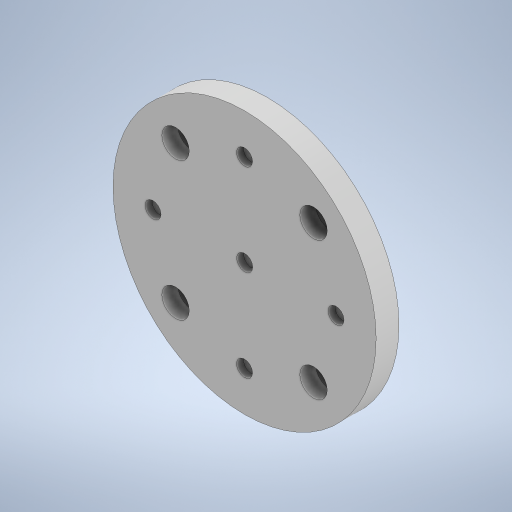
# Autodesk Inventor part: adaptor_spine_base
Saved by Autodesk Inventor 2024 (Build 280153000, 153)
## iProperties
Created: 2024-05-24
Part Number: adaptor_spine_base
Material: Generic
Document SubType Name: Modeling
Designer: maint
Density: 1 g/cm^3
Appearance: Default
Author: maint
Autodesk Inventor part; units mm, degrees
ref_plane "YZ Plane" through (0, 0, 0) normal (1, 0, 0) x (0, 1, 0)
ref_plane "XZ Plane" through (0, 0, 0) normal (0, 1, 0) x (-1, 0, 0)
ref_plane "XY Plane" through (0, 0, 0) normal (0, 0, 1) x (1, 0, 0)
sketch "Sketch1" plane through (0, 0, 0) normal (0, 0, 1) x (1, 0, 0)
  line L0 (40, -40) -> (-40, -40)
  line L1 (-40, -40) -> (-40, 40)
  line L2 (-40, 40) -> (40, 40)
  line L3 (40, 40) -> (40, -40)
  line L4 (40, -40) -> (-40, 40) construction
  line L5 (-40, -40) -> (40, 40) construction
  circle A0 centre (0, 0) radius 57.5
  dimension "d0" = 80
  dimension "d72" = 115
  constraints: 12 end point, 2 midpoint, 2 parallel, 2 perpendicular, 1 centre point, 1 coincident, 1 horizontal
  measures "d0" distance of L1.end L2.end
  measures "d72" diameter of A0
extrude "Extrusion1" add sketch "Sketch1" along normal blind 10 contours L0 L1 L2 L3 | A0
sketch "Sketch2" plane through (0, 0, 0) normal (0, 0, -1) x (-1, 0, 0)
  arc A0 (40, 37) -> (37, 40) centre (37, 37) ccw
  line L0 (30.15, -30.15) -> (-30.15, -30.15)
  line L1 (-30.15, -30.15) -> (-30.15, 30.15)
  line L2 (-30.15, 30.15) -> (30.15, 30.15)
  line L3 (30.15, 30.15) -> (30.15, -30.15)
  line L4 (30.15, -30.15) -> (-30.15, 30.15) construction
  line L5 (-30.15, -30.15) -> (30.15, 30.15) construction
  circle A1 centre (-30.15, 30.15) radius 4.75
  circle A2 centre (30.15, 30.15) radius 4.75
  circle A3 centre (30.15, -30.15) radius 4.75
  circle A4 centre (-30.15, -30.15) radius 4.75
  point P0 (0, 0)
  point P1 (39.1213, 39.1213)
  dimension "d32" = 60.3
  dimension "d33" = 9.5
  constraints: 12 end point, 5 centre point, 4 coincident, 3 equal radius, 3 point on circle, 2 midpoint, 2 parallel, 2 perpendicular, 1 horizontal
  measures "d32" distance of L1.end L2.end
  measures "d33" diameter of A2
hole "Hole3" at (30.15, -30.15, 0) at (30.15, 30.15, 0) at (-30.15, 30.15, 0) at (-30.15, -30.15, 0) direction (0, 0, 1) diameter 6.6 end through all
sketch "Sketch3" plane through (0, 0, 0) normal (0, 0, -1) x (-1, 0, 0)
  circle A0 centre (0, 0) radius 40
  circle A1 centre (0, 40) radius 2.5
  circle A2 centre (40, 0) radius 2.5
  circle A3 centre (0, -40) radius 2.5
  circle A4 centre (-40, 0) radius 2.5
  circle A5 centre (-0.0779, 0.0489) radius 2.5
  dimension "d12" = 5
  dimension "d60" = 80
  dimension "d74" = 5
  constraints: 6 centre point, 4 point on circle, 3 equal radius
  measures "d12" diameter of A1
  measures "d60" diameter of A0
  measures "d74" diameter of A5
hole "Hole1" at (40, 0, 0) at (0, 40, 0) at (0, -40, 0) at (-40, 0, 0) at (0.0779, 0.0489, 0) direction (0, 0, 1) diameter 7 end through all
sketch "Sketch8" plane through (0, 0, 0) normal (0, 0, -1) x (-1, 0, 0)
  circle A0 centre (0, 0) radius 40
  circle A1 centre (0, 40) radius 12.0233
  circle A2 centre (40, 0) radius 12.001
  circle A3 centre (-40, 0) radius 12.185
  circle A4 centre (0, -40) radius 12.001
  circle A5 centre (-0.3746, -0.3656) radius 12.0233
  dimension "d61" = 80
  constraints: 6 centre point, 4 point on circle
  measures "d61" diameter of A0
hole "Hole4" at (-40, 0, 0) at (0, 40, 0) at (40, 0, 0) at (0, -40, 0) at (0.3746, -0.3656, 0) direction (0, 0, 1) diameter 20 depth 7
sketch "Sketch10" plane through (0, 0, 10) normal (0, 0, 1) x (1, 0, 0)
  circle A0 centre (30.15, 30.15) radius 3.3 projected
  circle A1 centre (30.15, 30.15) radius 6
  circle A2 centre (-30.15, 30.15) radius 3.3 projected
  circle A3 centre (-30.15, 30.15) radius 6
  circle A4 centre (-30.15, -30.2444) radius 6
  circle A5 centre (30.15, -30.2444) radius 6
  point P0 (0, 0)
  dimension "d63" = 12
  constraints: 4 centre point, 3 equal radius, 2 coincident
  measures "d63" diameter of A1
hole "Hole5" at (-30.15, -30.2444, 10) at (30.15, -30.2444, 10) at (30.15, 30.15, 10) at (-30.15, 30.15, 10) direction (0, 0, -1) diameter 12 depth 7
body "Solid1"
